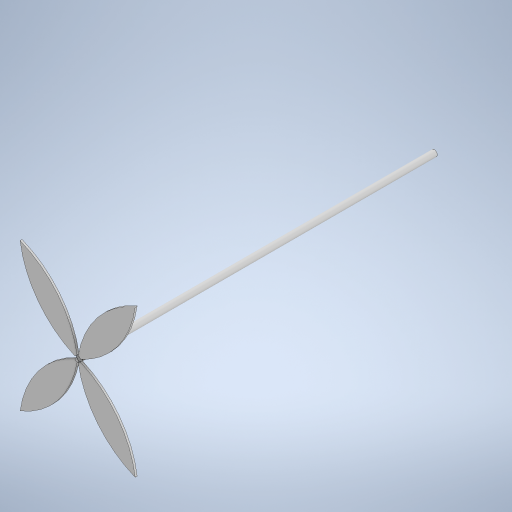
# Autodesk Inventor part: ranpro
Saved by Autodesk Inventor 2024 (Build 280153000, 153)
## iProperties
Created: 2024-09-09
Part Number: ranpro
Material: Generic
Document SubType Name: Modeling
Designer: srira
Density: 1 g/cm^3
Appearance: Default
Author: srira
Autodesk Inventor part; units mm, degrees
ref_plane "YZ Plane" through (0, 0, 0) normal (1, 0, 0) x (0, 1, 0)
ref_plane "XZ Plane" through (0, 0, 0) normal (0, 1, 0) x (-1, 0, 0)
ref_plane "XY Plane" through (0, 0, 0) normal (0, 0, 1) x (1, 0, 0)
sketch "Sketch1" plane through (0, 0, 0) normal (0, 0, 1) x (1, 0, 0)
  circle A0 centre (0, 0) radius 7.5
  circle A1 centre (0, 0) radius 8
  dimension "d0" = 15
  dimension "d1" = 16
  constraints: 2 centre point, 2 coincident
  measures "d0" diameter of A0
  measures "d1" diameter of A1
extrude "Extrusion1" add sketch "Sketch1" along normal blind 910
sketch "Sketch2" plane through (0, 0, 910) normal (0, 0, 1) x (1, 0, 0)
  circle A0 centre (0, 0) radius 8 projected
  arc A1 (147.6186, 189.232) -> (0, 0) centre (237.689, -33.2255) ccw
  arc A2 (0, 0) -> (147.6186, 189.232) centre (-90.0704, 222.4575) ccw
  line L0 (0, 102.2554) -> (0, 81.5536) construction
  arc A3 (0, 0) -> (-147.6186, 189.232) centre (-237.689, -33.2255) ccw
  arc A4 (-147.6186, 189.232) -> (0, 0) centre (90.0704, 222.4575) ccw
  line L1 (-25.0323, 0) -> (60.2591, 0) construction
  arc A5 (0, 0) -> (147.6186, -189.232) centre (237.689, 33.2255) ccw
  arc A6 (147.6186, -189.232) -> (0, 0) centre (-90.0704, -222.4575) ccw
  arc A7 (-147.6186, -189.232) -> (0, 0) centre (-237.689, 33.2255) ccw
  arc A8 (0, 0) -> (-147.6186, -189.232) centre (90.0704, -222.4575) ccw
  point P0 (-7.3642, -3.1255)
  point P1 (-1.2394, -7.9034)
  point P2 (7.3642, -3.1255)
  point P3 (1.2394, -7.9034)
  point P4 (7.3642, 3.1255)
  point P5 (1.2394, 7.9034)
  point P6 (-7.3642, 3.1255)
  point P7 (-1.2394, 7.9034)
  dimension "d17" = 240
  dimension "d18" = 240
  dimension "d19" = 240
  constraints: 16 point on circle, 9 symmetric about line, 8 centre point, 4 end point, 1 horizontal, 1 vertical, 6 other
  measures "d17" distance of A0.centre A1.start
  measures "d18" radius of A1
  measures "d19" radius of A2
extrude "Extrusion3" add sketch "Sketch2" along normal blind 5 contours A0 A1 A2 | A6 A5 A0 | A0 A4 A3 | A7 A8 A0 picked at (63.8091, 98.9231) picked at (80.4206, -85.9646) picked at (-80.4206, 85.9646) picked at (-63.8091, -98.9231)
body "Solid1"
